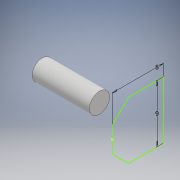
# Autodesk Inventor part: flat_cranial_window_stabilizer_Apr0119
Saved by Autodesk Inventor 2018 (Build 220112000, 112)
## iProperties
Created: 2018-06-11
Part Number: flat_cranial_window_stabilizer_Apr0119
Material: Generic
Document SubType Name: Modeling
Designer: McCormick Lab
Density: 1 g/cm^3
Appearance: Default
Author: McCormick Lab
Autodesk Inventor part; units mm, degrees
ref_plane "YZ Plane" through (0, 0, 0) normal (1, 0, 0) x (0, 1, 0)
ref_plane "XZ Plane" through (0, 0, 0) normal (0, 1, 0) x (-1, 0, 0)
ref_plane "XY Plane" through (0, 0, 0) normal (0, 0, 1) x (1, 0, 0)
sketch "Sketch1" plane through (0, 0, 0) normal (0, 1, 0) x (-1, 0, 0)
  arc A0 (0, -5) -> (0, 5) centre (0, 0) ccw
  line L0 (0, 5) -> (0, -5)
  dimension "d0" = 10
  constraints: 2 end point, 2 point on circle, 1 centre point, 1 coincident, 1 vertical
  measures "d0" diameter of A0
extrude "Extrusion1" add sketch "Sketch1" along normal blind 10
sketch "Sketch2" plane through (0, 0, 0) normal (1, 0, 0) x (0, 1, 0)
  line L0 (8.0172, -4.5) -> (8.0172, 4.5)
  line L1 (8.0172, 4.5) -> (2.5172, 4.5)
  line L2 (2.5172, -4.5) -> (0.0172, -2)
  line L3 (2.5172, 4.5) -> (0.0172, 2)
  line L4 (0.0172, -2) -> (0.0172, 2)
  line L5 (8.0172, -4.5) -> (2.5172, -4.5)
  point P0 (0, 0)
  dimension "d3" = 9
  dimension "d4" = 8
  constraints: 12 end point
  measures "d3" distance of L0.start L1.start
  measures "d4" distance between parallel lines of L0 L4
sketch "Sketch3" plane through (0, 0, 0) normal (1, 0, 0) x (0, 1, 0)
  line L0 (0, 2) -> (3, 5)
  arc A0 (3, 5) -> (0, 2) centre (1, 4) ccw
  line L1 (0, -2) -> (4, -6)
  arc A1 (0, -2) -> (4, -6) centre (1.75, -4.25) ccw
  line L2 (8.0325, 5) -> (11, 5)
  line L3 (11, 5) -> (11, -6)
  line L4 (11, -6) -> (8.0325, -6)
  line L5 (8.0325, -6) -> (8.0325, 5)
  line L6 (2.4911, 4.4911) -> (5, 7)
  line L7 (2.4911, 4.4911) -> (8.0325, 4.4911)
  arc A2 (8.0325, 4.4911) -> (5, 7) centre (7, 6.3303) ccw
  line L8 (2.4911, -4.4911) -> (8.5706, -4.4911)
  arc A3 (2.4911, -4.4911) -> (8.5706, -4.4911) centre (5.5309, -7.5041) ccw
  point P0 (0, 0)
  constraints: 18 end point, 8 point on circle, 4 centre point, 3 point on line, 2 horizontal, 2 parallel, 2 perpendicular
extrude "Extrusion2" cut sketch "Sketch3" against normal through all
sketch "Sketch4" plane through (0, 0, 0) normal (0, 1, 0) x (-1, 0, 0)
  arc A0 (1.0726, -4.4911) -> (1.0726, 4.4911) centre (-1.125, 0) ccw
  arc A1 (1.0726, 4.4911) -> (1.0726, -4.4911) centre (-0.4517, 0) ccw
  point P0 (0, 0)
  point P1 (2.1976, -4.4911)
  point P2 (2.1976, 4.4911)
  dimension "d9" = 1.125
  dimension "d10" = 1.125
  constraints: 4 point on circle, 2 centre point
  measures "d9" distance of point (2.198, 4.491) A0.end
  measures "d10" distance of point (2.198, -4.491) A0.start
extrude "Extrusion3" cut sketch "Sketch4" along normal through all both and the other way through all
sketch "Sketch5" plane through (0, 0, 0) normal (1, 0, 0) x (0, 1, 0)
  line L0 (1.6, -1.2445) -> (1.6, 1.1555)
  line L1 (6.4325, 2.6911) -> (3.1125, 2.6911)
  line L2 (6.4325, -2.6911) -> (6.4325, 2.6911)
  line L3 (6.4325, -2.6911) -> (3.1125, -2.6911)
  line L4 (0, 2) -> (0, -2) projected
  line L5 (8.0325, 4.4911) -> (8.0325, -4.4911) projected
  line L6 (0, 2) -> (2.4911, 4.4911) projected
  line L7 (2.4911, 4.4911) -> (8.0325, 4.4911) projected
  line L8 (8.0325, 4.4911) -> (8.0325, -4.4911) projected
  line L9 (8.0325, -4.4911) -> (2.4911, -4.4911) projected
  line L10 (2.4911, -4.4911) -> (0, -2) projected
  line L11 (0, 2) -> (0, -2) projected
  line L12 (1.6, 1.1555) -> (3.1125, 2.6911)
  line L13 (1.6, -1.2445) -> (3.1125, -2.6911)
  line L14 (1.6, 4.6579) -> (1.6, -5.3823)
  arc A0 (1.6, 4.6579) -> (1.6, -5.3823) centre (3.2437, -0.3622) ccw
  line L15 (1.6, 1.1555) -> (5.4757, 5.0906)
  line L16 (1.6, 1.1555) -> (1.6, 7.5999)
  arc A1 (5.4757, 5.0906) -> (1.6, 7.5999) centre (3.8837, 6.8794) ccw
  line L17 (3.1125, 2.6911) -> (12.4034, 2.6911)
  line L18 (3.1125, 2.6911) -> (8.5318, 8.1936)
  arc A2 (12.4034, 2.6911) -> (8.5318, 8.1936) centre (8.3272, 3.9364) ccw
  line L19 (6.4325, 2.6911) -> (13.6333, 2.6911)
  line L20 (6.4325, 2.6911) -> (6.4325, -9.3636)
  arc A3 (6.4325, -9.3636) -> (13.6333, 2.6911) centre (6.37, -1.1482) ccw
  line L21 (6.4325, -2.6911) -> (6.4325, -11.5775)
  line L22 (6.4325, -2.6911) -> (3.1125, -2.6911)
  line L23 (3.1125, -2.6911) -> (3.2437, -12.8567)
  arc A4 (3.2437, -12.8567) -> (6.4325, -9.3636) centre (5.6123, -11.8169) ccw
  line L24 (1.6, -1.2445) -> (1.6, -8.2222)
  line L25 (1.6, -1.2445) -> (3.1125, -2.6911)
  line L26 (3.1125, -2.6911) -> (3.1946, -9.0574)
  arc A5 (1.6, -8.2222) -> (3.1946, -9.0574) centre (2.6381, -8.1801) ccw
  point P0 (0, 0)
  dimension "d16" = 1.6
  dimension "d18" = 1.6
  dimension "d21" = 1.8
  dimension "d23" = 1.8
  dimension "d24" = 2.4
  dimension "d26" = 3.32
  dimension "d27" = 3.32
  constraints: 38 end point, 12 point on circle, 6 centre point, 4 point on line, 3 vertical, 2 collinear, 2 horizontal
  measures "d16" distance between parallel lines of L4 L0
  measures "d18" distance between parallel lines of L5 L2
  measures "d21" distance between parallel lines of L7 L1
  measures "d23" distance between parallel lines of L9 L3
  measures "d24" distance of L0.start L0.end
  measures "d26" distance of L1.start L1.end
  measures "d27" distance of L2.start L3.end
extrude "Extrusion4" cut sketch "Sketch5" against normal through all contours L14 L10 L4 L6 L0 | L13 L23 L9 L10 L14 | L14 L6 L7 L15 L12 | L3 L20 L9 L23 | L14 A0 L6 L4 L10 | L10 L9 L23 A5 L24 L14 | L15 L7 L5 L17 L1 | L14 L16 A1 L15 L7 L6 | L2 L17 L5 L9 L20 | L9 L20 A4 L23 | L15 L18 A2 L17 L5 L7 | L9 L5 L17 L19 A3 L20
sketch "Sketch6" plane through (0, 0, 0) normal (1, 0, 0) x (0, 1, 0)
  circle A0 centre (4, 0) radius 1.575
  line L0 (1.6, -1.2445) -> (1.6, 1.1555) projected
  point P0 (0, 0)
  dimension "d31" = 3.15
  dimension "d32" = 2.4
  constraints: 1 centre point
  measures "d31" diameter of A0
  measures "d32" distance from line of L0 A0.centre
extrude "Extrusion5" add sketch "Sketch6" against normal blind 15
sketch "Sketch7" plane through (0, 0, 0) normal (0, 1, 0) x (-1, 0, 0)
  arc A0 (3.089, -2.6911) -> (3.7176, -1.2445) centre (-1.125, 0) ccw projected
  arc A1 (3.7397, 1.1555) -> (3.089, 2.6911) centre (-1.125, 0) ccw projected
  arc A2 (3.7176, -1.2445) -> (3.7397, 1.1555) centre (-1.125, 0) ccw
  arc A3 (3.089, 2.6911) -> (3.089, -2.6911) centre (1.8078, 0) ccw
  point P0 (0, 0)
  constraints: 4 point on circle, 2 centre point
extrude "Extrusion6" cut sketch "Sketch7" along normal through all
sketch "Sketch8" plane through (-15, 4, 0) normal (-1, 0, 0) x (0, 0, 1)
  circle A0 centre (0, 0) radius 0.5375
  point P0 (0, -4)
  dimension "d37" = 1.075
  constraints: 1 centre point
  measures "d37" diameter of A0
extrude "Extrusion7" cut sketch "Sketch8" against normal blind 7
sketch "Sketch9" plane through (0, 0, 0) normal (0, 1, 0) x (-1, 0, 0)
  line L0 (6, 3) -> (2, 3)
  line L1 (2, 3) -> (2, -3)
  line L2 (2, -3) -> (6, -3)
  line L3 (6, -3) -> (6, 3)
  point P0 (0, 0)
  constraints: 8 end point, 2 parallel, 1 horizontal, 1 perpendicular
extrude "Extrusion8" cut sketch "Sketch9" along normal through all both and the other way through all
body "Solid1"
